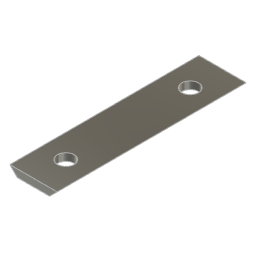
vrail spacer m3 (Autodesk Fusion 360 design; units mm, degrees)
Autodesk Fusion 360 part; units mm, degrees
sketch "Sketch1" plane through (0, 0, 0) normal (0, 1, 0) x (1, 0, 0)
  line L0 (-3.25, 0) -> (3.25, 0)
  line L1 (-4.75, -1.5) -> (4.75, -1.5)
  line L2 (0, -1.5) -> (0, 0) construction
  line L3 (-3.25, 0) -> (-4.75, -1.5)
  line L4 (3.25, 0) -> (4.75, -1.5)
  dimension "d1" = 6.5
  dimension "d2" = 9.5
  dimension "d3" = 45
  constraint horizontal L0
  constraint midpoint L0 L2.end
  constraint coincident L2.end origin
  constraint horizontal L1
  constraint midpoint L1 L2.start
  constraint vertical L2
  measures "d1" distance of L0.start L0.end
  measures "d2" distance of L1.start L1.end
  measures "d3" angle of L1 L3
extrude "Extrude1" add sketch "Sketch1" along normal blind 38
sketch "Sketch2" plane through (0, 0, 1.5) normal (0, 0, 1) x (-1, 0, 0)
  line L0 (4.75, 0) -> (-4.75, 0)
  line L1 (-4.75, 0) -> (-4.75, -38)
  line L2 (-4.75, -38) -> (4.75, -38)
  line L3 (4.75, -38) -> (4.75, 0)
  line L4 (0, 0) -> (0, -38) construction
  point P0 (0, -31.5)
  point P1 (0, -6.5)
  dimension "d6" = 25
  dimension "d7" = 6.5
  constraint coincident L4.start origin
  constraint midpoint L2 L4.end
  constraint coincident L4 P0
  constraint coincident L4 P1
  measures "d6" distance of P0 P1
  measures "d7" distance of L2 P0
hole "Hole1" at (0, 31.5, 1.5) at (0, 6.5, 1.5) direction (0, 0, -1) diameter 3.4 depth 16 tip angle 118
